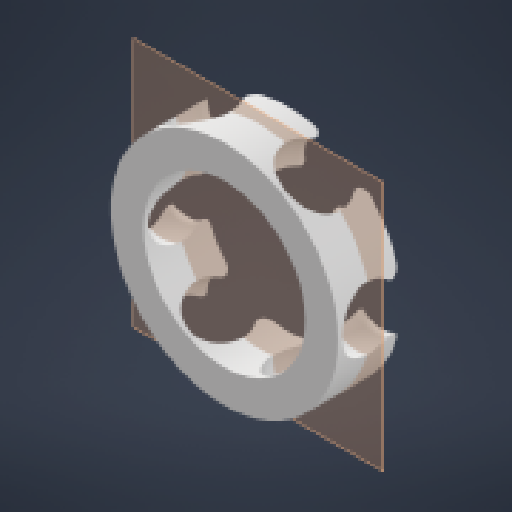
# Autodesk Inventor part: Spacer
Saved by Autodesk Inventor 2023 (Build 270158000, 158)
## iProperties
Created: 2023-02-24
Part Number: Spacer
Material: Generic
Document SubType Name: Modeling
Designer: izack
Density: 1 g/cm^3
Appearance: Default
Author: izack
Autodesk Inventor part; units mm, degrees
ref_plane "YZ Plane" through (0, 0, 0) normal (1, 0, 0) x (0, 1, 0)
ref_plane "XZ Plane" through (0, 0, 0) normal (0, 1, 0) x (-1, 0, 0)
ref_plane "XY Plane" through (0, 0, 0) normal (0, 0, 1) x (1, 0, 0)
sketch "Sketch1" plane through (0, 0, 0) normal (0, 0, 1) x (1, 0, 0)
  circle A0 centre (-8.25, 0) radius 4 projected
  circle A1 centre (-8.25, 0) radius 5 projected
  circle A2 centre (-8.25, 0) radius 8.25 projected
  circle A3 centre (-8.25, 0) radius 5.5
  circle A4 centre (-8.25, 0) radius 7.75
  point P0 (0, 0)
  dimension "d0" = 0.5
  dimension "d1" = 0.5
  constraints: 2 centre point, 1 horizontal alignment
  measures "d0" radial gap between concentric circles of A1 A3
extrude "Extrusion1" add sketch "Sketch1" against normal blind 4.5 contours A4
ref_plane "Work Plane1" through (-8.25, 0, -2.5) normal (0, 0, 1) x (1, 0, 0)
sketch "Sketch2" plane through (-8.25, 0, -2.5) normal (0, 0, 1) x (1, 0, 0)
  circle A0 centre (0, 0) radius 7.75 projected
  line L0 (-7.75, 0) -> (-5.5, 0)
  circle A1 centre (0, 0) radius 5.5 projected
  circle A2 centre (-6.625, 0) radius 2.3
  line L1 (-8.925, 0) -> (-4.325, 0)
  point P0 (8.25, 0)
  dimension "d5" = 4.6
  constraints: 4 end point, 2 horizontal, 2 horizontal alignment, 2 point on circle, 1 centre point, 1 midpoint, 2 other
  measures "d5" diameter of A2
revolve "Revolution1" cut sketch "Sketch2" angle 360 about axis through (-17.175, 0, -2.5) along (1, 0, 0) picked at (-8.1082, -0.4246) picked at (-6.497, -1.6514) picked at (-5.1163, -0.3748) contours A2 L1 A0 | A0 L0 A1 A2 | A1 L1 A2
fillet "Fillet1" radius 0.5 2 edges at (-14.8616, -1.1357, -4.5) (-14.8616, 1.1357, -4.5)
pattern_circular "Circular Pattern1" count 6 over 360 about axis through (-8.25, 0, 0) along (0, 0, -1) of "Revolution1", "Fillet1"
sketch "Sketch3" plane through (-8.25, 0, 0) normal (0, 0, 1) x (1, 0, 0)
  circle A0 centre (0, 0) radius 7.75 projected
  circle A1 centre (0, 0) radius 5.5 projected
  point P0 (8.25, 0)
extrude "Extrusion2" cut sketch "Sketch3" against normal blind 0.2
body "Solid1"
